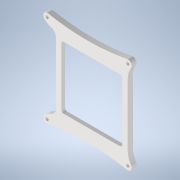
# Autodesk Inventor part: jetson_deckel
Saved by Autodesk Inventor 2021.3 (Build 253353010, 353A)
## iProperties
Created: 2021-07-27
Part Number: jetson_deckel
Material: Generisch
Document SubType Name: Modeling
Designer: Markus
Density: 1 g/cm^3
Appearance: Vorgabe
Author: Markus
Autodesk Inventor part; units mm, degrees
ref_plane "YZ Plane" through (0, 0, 0) normal (1, 0, 0) x (0, 1, 0)
ref_plane "XZ Plane" through (0, 0, 0) normal (0, 1, 0) x (-1, 0, 0)
ref_plane "XY Plane" through (0, 0, 0) normal (0, 0, 1) x (1, 0, 0)
sketch "Skizze1" plane through (0, 0, 0) normal (0, 0, 1) x (1, 0, 0)
  line L0 (46.5, 52.5) -> (-46.5, 52.5) projected
  line L1 (-46.5, 52.5) -> (-46.5, -52.5) projected
  line L2 (-46.5, -52.5) -> (46.5, -52.5) projected
  line L3 (46.5, -52.5) -> (46.5, 52.5) projected
  circle A0 centre (49, -60.25) radius 5.3 projected
  circle A1 centre (49, -60.25) radius 2 projected
  circle A2 centre (49, 60.25) radius 5.3 projected
  circle A3 centre (49, 60.25) radius 2 projected
  circle A4 centre (-61, 60.25) radius 5.3 projected
  circle A5 centre (-61, 60.25) radius 2 projected
  circle A6 centre (-61, -60.25) radius 5.3 projected
  circle A7 centre (-61, -60.25) radius 2 projected
  line L4 (49, 60.25) -> (-61, 60.25) construction
  line L5 (49, -60.25) -> (-61, -60.25) construction
  arc A8 (-59.9879, 65.4525) -> (47.9879, 65.4525) centre (-6, 342.9774) ccw
  arc A9 (47.9879, -65.4525) -> (-59.9879, -65.4525) centre (-6, -342.9774) ccw
  line L6 (-41.5, 39.5) -> (-41.5, -39.5)
  line L7 (41.5, -39.5) -> (41.5, 39.5)
  line L8 (38.5, 42.5) -> (-38.5, 42.5)
  line L9 (38.5, -42.5) -> (-38.5, -42.5)
  arc A10 (41.5, 39.5) -> (38.5, 42.5) centre (38.5, 39.5) ccw
  arc A11 (38.5, -42.5) -> (41.5, -39.5) centre (38.5, -39.5) ccw
  arc A12 (-41.5, -39.5) -> (-38.5, -42.5) centre (-38.5, -39.5) ccw
  arc A13 (-38.5, 42.5) -> (-41.5, 39.5) centre (-38.5, 39.5) ccw
  line L10 (-49, 42.5) -> (-49, -42.5)
  line L11 (49, 42.5) -> (49, -42.5)
  arc A14 (-64.7477, 56.5023) -> (-55.7, 51.2598) centre (-50.3799, 70.8701) ccw
  arc A15 (-49, 42.5) -> (-55.7, 51.2598) centre (-58.0765, 42.5) ccw
  arc A16 (-59.9879, 65.4525) -> (-64.7477, 56.5023) centre (-61, 60.25) ccw
  arc A17 (-55.7, -51.2598) -> (-64.7477, -56.5023) centre (-50.3799, -70.8701) ccw
  arc A18 (-55.7, -51.2598) -> (-49, -42.5) centre (-58.0765, -42.5) ccw
  arc A19 (-64.7477, -56.5023) -> (-59.9879, -65.4525) centre (-61, -60.25) ccw
  arc A20 (53.4323, 57.344) -> (49, 42.5) centre (76.0729, 42.5) ccw
  arc A21 (49, -42.5) -> (53.4323, -57.344) centre (76.0729, -42.5) ccw
  arc A22 (53.4323, 57.344) -> (47.9879, 65.4525) centre (49, 60.25) ccw
  arc A23 (47.9879, -65.4525) -> (53.4323, -57.344) centre (49, -60.25) ccw
  circle A24 centre (49, -60.25) radius 2.25
  circle A25 centre (-61, -60.25) radius 2.25
  circle A26 centre (-61, 60.25) radius 2.25
  circle A27 centre (49, 60.25) radius 2.25
  point P0 (-6, 60.25)
  point P1 (-6, -60.25)
  point P2 (-55.7, 60.25)
  dimension "d34" = 5
  dimension "d35" = 5
  dimension "d36" = 10
  dimension "d37" = 10
  dimension "d38" = 3
  dimension "d39" = 2.5
  dimension "d40" = 2.5
  dimension "d41" = 45
  dimension "d42" = 45
  dimension "d43" = 0.25
  dimension "d44" = 0.25
  dimension "d45" = 0.25
  dimension "d46" = 0.25
  constraints: 43 point on circle, 26 tangent, 20 centre point, 16 end point, 5 equal radius, 4 horizontal alignment, 2 horizontal, 2 midpoint, 2 parallel, 2 vertical, 2 vertical alignment, 1 point on line
  measures "d34" distance between parallel lines of L3 L7
  measures "d35" distance between parallel lines of L1 L6
  measures "d36" distance between parallel lines of L0 L8
  measures "d37" distance between parallel lines of L2 L9
  measures "d38" radius of A10
  measures "d39" distance between parallel lines of L3 L11
  measures "d40" distance between parallel lines of L1 L10
  measures "d43" radial gap between concentric circles of A1 A24
  measures "d44" radial gap between concentric circles of A7 A25
  measures "d45" radial gap between concentric circles of A5 A26
  measures "d46" radial gap between concentric circles of A27 A3
extrude "Extrusion1" add sketch "Skizze1" along normal blind 5 contours L3 L2 L1 L0 | A0 | A0 A9 A6 A17 A18 L10 A15 A14 A4 A8 A2 A20 L11 A21 | A6 | A2 | A4
sketch "Skizze2" plane through (0, 0, 0) normal (0, 0, -1) x (-1, 0, 0)
  arc A0 (59.9879, -65.4525) -> (64.7477, -56.5023) centre (61, -60.25) ccw projected
  arc A1 (64.7477, 56.5023) -> (59.9879, 65.4525) centre (61, 60.25) ccw projected
  line L0 (-46.5, 52.5) -> (46.5, 52.5) projected
  line L1 (46.5, 52.5) -> (46.5, -52.5) projected
  line L2 (46.5, -52.5) -> (-46.5, -52.5) projected
  line L3 (-46.5, -52.5) -> (-46.5, 52.5) projected
  line L4 (47, 53) -> (-47, 53)
  line L5 (-47, 53) -> (-47, -53)
  line L6 (-47, -53) -> (47, -53)
  line L7 (47, -53) -> (47, 53)
  arc A2 (-47.9879, 65.4525) -> (-53.4323, 57.344) centre (-49, 60.25) ccw projected
  arc A3 (-47.9879, 65.4525) -> (59.9879, 65.4525) centre (6, 342.9774) ccw projected
  arc A4 (-49, 42.5) -> (-53.4323, 57.344) centre (-76.0729, 42.5) ccw projected
  line L8 (-49, -42.5) -> (-49, 42.5) projected
  arc A5 (-53.4323, -57.344) -> (-49, -42.5) centre (-76.0729, -42.5) ccw projected
  arc A6 (-53.4323, -57.344) -> (-47.9879, -65.4525) centre (-49, -60.25) ccw projected
  arc A7 (59.9879, -65.4525) -> (-47.9879, -65.4525) centre (6, -342.9774) ccw projected
  arc A8 (64.7477, -56.5023) -> (55.7, -51.2598) centre (50.3799, -70.8701) ccw projected
  arc A9 (49, -42.5) -> (55.7, -51.2598) centre (58.0765, -42.5) ccw projected
  line L9 (49, 42.5) -> (49, -42.5) projected
  arc A10 (55.7, 51.2598) -> (49, 42.5) centre (58.0765, 42.5) ccw projected
  arc A11 (55.7, 51.2598) -> (64.7477, 56.5023) centre (50.3799, 70.8701) ccw projected
  circle A12 centre (61, 60.25) radius 2.25 projected
  circle A13 centre (61, -60.25) radius 2.25 projected
  circle A14 centre (-49, -60.25) radius 2.25 projected
  circle A15 centre (-49, 60.25) radius 2.25 projected
  point P0 (0, 0)
  dimension "d30" = 0.5
  constraints: 8 end point, 3 other
  measures "d30" distance between parallel lines of L0 L4
extrude "Extrusion2" add sketch "Skizze2" along normal blind 2 contours A7 A6 A5 L8 A4 A2 A3 A1 A11 A10 L9 A9 A8 A0 | L7 L6 L5 L4
equation "\"d35\" = d34"
equation "\"d37\" = d36"
equation "\"d40\" = d39"
equation "\"d44\" = d43"
equation "\"d45\" = d43"
equation "\"d46\" = d43"
